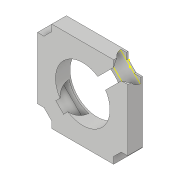
# Autodesk Inventor part: 20_Cube_Insert_Lens_Cylindrical_v3
Saved by Autodesk Inventor 2019.4 (Build 234330000, 330)
## iProperties
Created: 2019-07-24
Part Number: 20_Cube_Insert_Lens_Cylindrical_v3
Material: Generic
Document SubType Name: Modeling
Designer: marsikovabarbora
Density: 1 g/cm^3
Appearance: Default
Author: marsikovabarbora
Autodesk Inventor part; units mm, degrees
ref_plane "YZ Plane" through (0, 0, 0) normal (1, 0, 0) x (0, 1, 0)
ref_plane "XZ Plane" through (0, 0, 0) normal (0, 1, 0) x (-1, 0, 0)
ref_plane "XY Plane" through (0, 0, 0) normal (0, 0, 1) x (1, 0, 0)
sketch "Sketch1" plane through (0, 0, 0) normal (0, 0, 1) x (1, 0, 0)
  line L0 (21.5871, 13.6345) -> (17.0871, 18.1345) projected
  line L1 (17.0871, 18.1345) -> (-16.7129, 18.1345) projected
  line L2 (-16.7129, 18.1345) -> (-21.2129, 13.6345) projected
  line L3 (-21.0966, 13.6345) -> (-21.0966, -20.1655) projected
  line L4 (21.4709, -20.1655) -> (21.4709, 13.6345) projected
  line L5 (21.4709, -20.1655) -> (17.0871, -24.4078) projected
  line L6 (-16.7129, -24.4078) -> (17.0871, -24.4078) projected
  line L7 (-16.7129, -24.4078) -> (-21.0966, -20.1655) projected
  line L8 (-24.7129, -28.1655) -> (-24.7129, 13.6345) construction
  line L9 (25.0871, -28.1655) -> (-24.7129, -28.1655) construction
  line L10 (25.0871, -28.1655) -> (25.0871, 13.6345) construction
  line L11 (17.0871, 21.6345) -> (-16.7129, 21.6345) construction
  line L12 (-21.0552, -20.0655) -> (-16.6129, -24.5078)
  line L13 (-16.6129, -24.5078) -> (-16.6129, -28.1655)
  line L14 (-16.6129, -28.1655) -> (17.0871, -28.1655)
  line L15 (25.0871, -20.0655) -> (21.4295, -20.0655)
  line L16 (25.0871, 13.5345) -> (25.0871, -20.0655)
  line L17 (21.4295, 13.5345) -> (25.0871, 13.5345)
  line L18 (21.4295, 13.5345) -> (16.9871, 17.9768)
  line L19 (16.9871, 17.9768) -> (16.9871, 21.6345)
  line L20 (16.9871, 21.6345) -> (-16.6129, 21.6345)
  line L21 (-16.6129, 21.6345) -> (-16.6129, 17.9768)
  line L22 (-16.6129, 17.9768) -> (-21.0552, 13.5345)
  line L23 (-24.7129, 13.5345) -> (-21.0552, 13.5345)
  line L24 (-24.7129, -20.0655) -> (-24.7129, 13.5345)
  line L25 (-21.0552, -20.0655) -> (-24.7129, -20.0655)
  line L26 (-12.3129, -23.2655) -> (12.6871, -23.2655) projected
  line L27 (12.6871, -23.2655) -> (12.6871, 16.7345) projected
  line L28 (-12.3129, 16.7345) -> (12.6871, 16.7345) projected
  line L29 (-12.3129, -23.2655) -> (-12.3129, 16.7345) projected
  line L30 (14.6871, -25.2655) -> (-14.3129, -25.2655) construction
  line L31 (-14.3129, -25.2655) -> (-14.3129, 18.7345) construction
  line L32 (-14.3129, 18.7345) -> (14.6871, 18.7345) construction
  line L33 (14.6871, 18.7345) -> (14.6871, -25.2655) construction
  line L34 (-17.3129, 21.7345) -> (17.6871, 21.7345) construction
  line L35 (17.6871, 21.7345) -> (17.6871, -28.2655) construction
  line L36 (17.6871, -28.2655) -> (-17.3129, -28.2655) construction
  line L37 (-17.3129, -28.2655) -> (-17.3129, 21.7345) construction
  line L38 (-14.3129, -23.2655) -> (-14.3129, -25.2655)
  line L39 (-14.3129, -25.2655) -> (14.6871, -25.2655)
  line L40 (14.6871, -25.2655) -> (14.6871, -20.0655)
  line L41 (14.6871, -20.0655) -> (17.6871, -20.0655)
  line L42 (17.6871, -20.0655) -> (17.6871, 13.5345)
  line L43 (17.6871, 13.5345) -> (14.6871, 13.5345)
  line L44 (14.6871, 13.5345) -> (14.6871, 18.7345)
  line L45 (14.6871, 18.7345) -> (-14.3129, 18.7345)
  line L46 (-14.3129, 18.7345) -> (-14.3129, 13.5345)
  line L47 (-14.3129, 13.5345) -> (-17.3129, 13.5345)
  line L48 (-17.3129, 13.5345) -> (-17.3129, -20.0655)
  line L49 (-17.3129, -20.0655) -> (-14.3129, -20.0655)
  line L50 (-14.3129, -20.0655) -> (-14.3129, -23.2655)
  line L51 (-16.6129, -28.1655) -> (17.0871, -28.1655)
  line L52 (16.9871, -28.1655) -> (16.9871, -24.3509)
  line L53 (16.9871, -24.3509) -> (21.2726, -20.0655)
  line L54 (21.2726, -20.0655) -> (21.4295, -20.0655)
  point P0 (14.2, -44.8454)
  point P1 (16.9871, 19.8057)
  dimension "d74" = 2
  dimension "d75" = 5
  dimension "d76" = 135
  constraints: 78 end point, 15 point on line, 7 horizontal, 5 vertical, 4 perpendicular, 3 collinear, 1 midpoint, 10 other
  measures "d74" distance between parallel lines of L26 L30
  measures "d75" distance between parallel lines of L29 L37
  measures "d76" angle of L52 L53
extrude "Extrusion1" add sketch "Sketch1" along normal blind 8 contours L19 L18 L17 L4 L15 L54 L53 L52 L6 L40 L41 L42 L43 L44 L1 | L1 L44 L45 L46 L21 L20 L19 | L44 L43 L42 L41 L40 L6 L38 L50 L49 L48 L47 L46 L1 | L1 L46 L45 L44 | L46 L47 L48 L49 L50 L38 L6 L12 L25 L3 L23 L22 L21 L1 | L17 L16 L15 L4 | L3 L25 L24 L23 | L40 L39 L38 L6 | L6 L52 L14 L13 L12 L38 L39 L40 | L29 L28 L27 L26
sketch "Skizze7" plane through (0, 0, 8) normal (0, 0, 1) x (1, 0, 0)
  line L0 (-21.0552, -20.0655) -> (-16.6129, -24.5078) projected
  line L1 (-16.6129, -24.5078) -> (-16.6129, -28.1655) projected
  line L2 (-16.6129, -28.1655) -> (16.9871, -28.1655) construction
  line L3 (16.9871, -28.1655) -> (16.9871, -24.3509) projected
  line L4 (16.9871, -24.3509) -> (21.2726, -20.0655) projected
  line L5 (21.2726, -20.0655) -> (25.0871, -20.0655) projected
  line L6 (25.0871, -20.0655) -> (25.0871, 13.5345) construction
  line L7 (25.0871, 13.5345) -> (21.4295, 13.5345) projected
  line L8 (21.4295, 13.5345) -> (16.9871, 17.9768) projected
  line L9 (16.9871, 17.9768) -> (16.9871, 21.6345) projected
  line L10 (16.9871, 21.6345) -> (-16.6129, 21.6345) construction
  line L11 (-16.6129, 21.6345) -> (-16.6129, 17.9768) projected
  line L12 (-16.6129, 17.9768) -> (-21.0552, 13.5345) projected
  line L13 (-21.0552, 13.5345) -> (-24.7129, 13.5345) projected
  line L14 (-24.7129, 13.5345) -> (-24.7129, -20.0655) construction
  line L15 (-24.7129, -20.0655) -> (-21.0552, -20.0655) projected
  line L16 (-16.8129, 21.8345) -> (17.1871, 21.8345) construction
  line L17 (17.1871, 21.8345) -> (17.1871, 18.0597)
  line L18 (17.1871, 18.0597) -> (21.5123, 13.7345)
  line L19 (21.5123, 13.7345) -> (25.2871, 13.7345)
  line L20 (25.2871, 13.7345) -> (25.2871, -20.2655) construction
  line L21 (25.2871, -20.2655) -> (21.3554, -20.2655)
  line L22 (21.3554, -20.2655) -> (17.1871, -24.4338)
  line L23 (17.1871, -24.4338) -> (17.1871, -28.3655)
  line L24 (17.1871, -28.3655) -> (-16.8129, -28.3655) construction
  line L25 (-16.8129, -28.3655) -> (-16.8129, -24.5907)
  line L26 (-16.8129, -24.5907) -> (-21.1381, -20.2655)
  line L27 (-21.1381, -20.2655) -> (-24.9129, -20.2655)
  line L28 (-24.9129, -20.2655) -> (-24.9129, 13.7345) construction
  line L29 (-24.9129, 13.7345) -> (-21.1381, 13.7345)
  line L30 (-21.1381, 13.7345) -> (-16.8129, 18.0597)
  line L31 (-16.8129, 18.0597) -> (-16.8129, 21.8345)
  line L32 (-21.0552, 13.5345) -> (-24.7129, 13.5345) projected
  line L33 (-24.7129, 13.5345) -> (-24.7129, 13.7345)
  line L34 (-16.6129, 21.6345) -> (-16.6129, 17.9768) projected
  line L35 (-16.6129, 21.6345) -> (-16.8129, 21.6345)
  line L36 (25.0871, -20.0655) -> (25.0871, 13.5345) projected
  line L37 (25.0871, 13.5345) -> (25.0871, 13.7345)
  line L38 (16.9871, 21.6345) -> (17.1871, 21.6345)
  line L39 (16.9871, -28.1655) -> (17.1871, -28.1655)
  line L40 (25.0871, -20.0655) -> (25.0871, -20.2655)
  line L41 (-16.6129, -28.1655) -> (-16.8129, -28.1655)
  line L42 (-24.7129, -20.0655) -> (-24.7129, -20.2655)
  dimension "d94" = 0.2
  constraints: 48 end point, 12 point on line, 4 perpendicular, 15 other
  measures "d94" distance between parallel lines of L10 L16
extrude "IM_offset" add sketch "Skizze7" against normal up to surface (8 mm away)
sketch "Sketch8" plane through (-1.6003, 36.8471, 0) normal (0.7071, 0.7071, 0) x (0.7071, -0.7071, 0)
  arc A0 (21.9778, -0.9777) -> (37.2778, -0.9777) centre (29.6278, -0.9777) ccw
  line L0 (21.9778, -0.9777) -> (37.2778, -0.9777) construction
  line L1 (21.9778, -0.9777) -> (37.2778, -0.9777) construction
  line L2 (21.9778, -0.9777) -> (37.2778, -0.9777)
  point P0 (27.1864, 0)
  point P1 (29.6278, -1.0154)
  dimension "d98" = 15.3
  dimension "d99" = 0
  dimension "d100" = 7.65
  constraints: 6 end point, 2 point on circle, 1 centre point, 1 collinear, 1 horizontal
  measures "d98" distance of L0.start L0.end
  measures "d99" distance between parallel lines of L0 L1
  measures "d100" radius of A0
extrude "Extrusion7" cut sketch "Sketch8" against normal blind 45 and the other way blind 22.5
sketch "Sketch9" plane through (0, 0, 8) normal (0, 0, 1) x (1, 0, 0)
  line L0 (17.1871, 21.6345) -> (-16.8129, 21.6345) projected
  line L1 (-24.7129, 13.7345) -> (-24.7129, -20.2655) projected
  line L2 (17.1871, -28.1655) -> (-16.8129, -28.1655) projected
  line L3 (25.0871, -20.0655) -> (25.0871, 13.7345) projected
  circle A0 centre (0.1871, -3.187) radius 27.0445
  circle A1 centre (0.1871, -3.187) radius 15
  line L4 (-16.8129, 21.6345) -> (-16.8129, 18.0597) projected
  line L5 (-16.8129, 18.0597) -> (-21.1381, 13.7345) projected
  line L6 (-21.1381, 13.7345) -> (-24.7129, 13.7345) projected
  line L7 (17.1871, -28.1655) -> (17.1871, -24.4338) projected
  line L8 (17.1871, -24.4338) -> (21.3554, -20.2655) projected
  line L9 (21.3554, -20.2655) -> (25.0871, -20.2655) projected
  line L10 (25.0871, -20.2655) -> (25.0871, -20.0655) projected
  line L11 (25.0871, 13.7345) -> (21.5123, 13.7345) projected
  line L12 (21.5123, 13.7345) -> (21.4956, 13.7512) projected
  line L13 (17.1871, 18.0597) -> (17.1871, 21.6345) projected
  line L14 (-21.1381, -20.2655) -> (-24.7129, -20.2655) projected
  line L15 (-16.8129, -24.5907) -> (-21.1381, -20.2655) projected
  line L16 (-16.8129, -28.1655) -> (-16.8129, -24.5907) projected
  line L17 (21.4956, 13.7512) -> (-10.3242, -18.0686) projected
  line L18 (-10.3242, -18.0686) -> (-14.6159, -13.7769) projected
  line L19 (-14.6159, -13.7769) -> (17.2039, 18.043) projected
  line L20 (17.2039, 18.043) -> (17.1871, 18.0597) projected
  point P0 (0, 0)
  dimension "d91" = 30
  constraints: 2 centre point, 1 coincident
  measures "d91" diameter of A1
extrude "Extrusion8" cut sketch "Sketch9" against normal through all contours L19 A1 | A1 L17 L19 | A1 L17
sketch "Sketch10" plane through (21.5123, 13.7345, 1.6478) normal (0.7071, 0.7071, 0) x (0, 0, -1)
  line L0 (-6.3522, 0.0237) -> (-6.3522, 6.0931) projected
  arc A0 (-6.3522, 0.0237) -> (0.6701, -4.5916) centre (0.6701, 3.0584) ccw projected
  line L1 (0.6701, 10.7084) -> (0.6701, -4.5916) projected
  arc A1 (0.6701, 10.7084) -> (-6.3522, 6.0931) centre (0.6701, 3.0584) ccw projected
  point P0 (1.6478, 5.4998)
body "Solid1"
